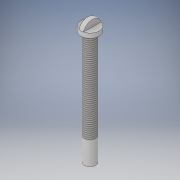
# Autodesk Inventor part: LeadScrew
Saved by Autodesk Inventor 2019 (Build 230136000, 136)
## iProperties
Created: 2019-08-02
Part Number: LeadScrew
Material: Generic
Document SubType Name: Modeling
Designer: aorfi
Density: 1 g/cm^3
Appearance: Default
Author: aorfi
Autodesk Inventor part; units mm, degrees
ref_plane "YZ Plane" through (0, 0, 0) normal (1, 0, 0) x (0, 1, 0)
ref_plane "XZ Plane" through (0, 0, 0) normal (0, 1, 0) x (-1, 0, 0)
ref_plane "XY Plane" through (0, 0, 0) normal (0, 0, 1) x (1, 0, 0)
sketch "Sketch1" plane through (0, 0, 0) normal (0, 1, 0) x (-1, 0, 0)
  circle A0 centre (0, 0) radius 2.5
  dimension "d0" = 5
  constraints: 1 centre point, 1 coincident
  measures "d0" diameter of A0
extrude "Extrusion1" add sketch "Sketch1" along normal mid plane 50
sketch "Sketch9" plane through (0, 25, 0) normal (0, 1, 0) x (1, 0, 0)
  circle A0 centre (0, 0) radius 4
  dimension "d56" = 8
  constraints: 1 centre point, 1 coincident
  measures "d56" diameter of A0
extrude "Extrusion2" add sketch "Sketch9" along normal blind 2
sketch "Sketch10" plane through (0, 0, 0) normal (1, 0, 0) x (0, 1, 0)
  line L0 (27, 4) -> (30, 4)
  line L1 (30, 4) -> (30, -4)
  line L2 (30, -4) -> (27, -4)
  line L3 (27, -4) -> (27, 4)
  line L4 (27, -4) -> (27, 4) projected
  point P0 (0, 0)
  point P1 (27, 0)
  point P2 (30, 0)
  dimension "d59" = 8
  dimension "d60" = 3
  constraints: 8 end point, 2 midpoint, 2 parallel, 1 collinear, 1 horizontal, 1 horizontal alignment, 1 perpendicular
  measures "d59" distance of L0.end L1.end
  measures "d60" distance of L1.end L2.end
extrude "Extrusion3" add sketch "Sketch10" along normal mid plane 2
sketch "Sketch11" plane through (0, 0, 0) normal (1, 0, 0) x (0, 1, 0)
  line L0 (32, 0) -> (32, -5)
  line L1 (27, -4) -> (27, -5)
  line L2 (27, -5) -> (32, -5)
  line L3 (30, 4) -> (30, -4) projected
  line L4 (32, 0) -> (30, 0)
  line L5 (-36.2, 0) -> (42.2, 0) projected
  line L6 (30, -4) -> (27, -4) projected
  arc A0 (27, -4) -> (30, 0) centre (25.8333, 0) ccw
  point P0 (0, 0)
  point P1 (27, 4)
  point P2 (31, 0)
  point P3 (27, -3.873)
  dimension "d65" = 5
  dimension "d68" = 2
  constraints: 8 end point, 2 midpoint, 2 perpendicular, 2 point on circle, 2 vertical, 1 centre point, 1 horizontal, 1 tangent
  measures "d65" distance of L0.start L0.end
  measures "d68" distance between parallel lines of L3 L0
revolve "Revolution5" cut sketch "Sketch11" angle 360 about axis through (0, -10, 0) along (0, 1, 0)
thread "Thread4" size "M5x0.8" class "6g" standard "ANSI Metric M Profile" length 40
equation "\"d23\" = 55deg"
equation "\"Sketch3_Pitch\" = 0.8"
equation "\"d44\" = 55deg"
equation "\"Sketch6_Pitch\" = 1.27"
body "Solid1"
